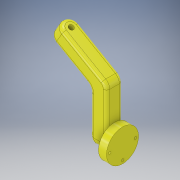
# Autodesk Inventor part: Link1
Saved by Autodesk Inventor 2019 (Build 230136000, 136)
## iProperties
Created: 2022-07-14
Part Number: Link1
Material: Generic
Document SubType Name: Modeling
Designer: zreik
Density: 1 g/cm^3
Appearance: Yellow
thickness: 10.000 mm
width: 10.000 mm
radius: 60.000 mm
Author: zreik
Autodesk Inventor part; units mm, degrees
sketch "Sketch1" plane through (0, 0, 0) normal (0, 0, 1) x (1, 0, 0)
  line L0 (54.744646, 0) -> (0, 0)
  line L1 (0, 0) -> (30, 51.961524)
  line L2 (44.744646, 0) -> (44.744646, 23.613249)
  line L3 (42.244646, 27.943376) -> (22.660998, 39.25)
  line L4 (54.744646, 0) -> (54.744646, 29.386751)
  line L5 (52.244646, 33.716878) -> (27.660998, 47.910254)
  arc A0 (44.744646, 23.613249) -> (42.244646, 27.943376) centre (39.744646, 23.613249) ccw
  arc A1 (54.744646, 29.386751) -> (52.244646, 33.716878) centre (49.744646, 29.386751) ccw
  line L6 (27.660998, 47.910254) -> (22.660998, 39.25)
  line L7 (27.660998, 47.910254) -> (52.244646, 33.716878)
  line L8 (22.660998, 39.25) -> (42.244646, 27.943376)
  line L9 (44.744646, 0) -> (54.744646, 0)
  line L10 (54.744646, 0) -> (54.744646, 29.386751)
  line L11 (44.744646, 0) -> (54.744646, 0)
  line L12 (54.744646, 0) -> (54.744646, 29.386751)
  line L13 (52.244646, 33.716878) -> (27.660998, 47.910254)
  line L14 (27.660998, 47.910254) -> (22.660998, 39.25)
  line L15 (22.660998, 39.25) -> (42.244646, 27.943376)
  line L16 (44.744646, 23.613249) -> (44.744646, 0)
  point P0 (25, 43.30127)
  point P1 (44.744646, 26.5)
  dimension "d0" = 60
  dimension "d35" = 10
  dimension "d37" = 10
  dimension "d38" = 0
  dimension "d39" = 0
  dimension "d41" = 26.5
  dimension "d42" = 25.5
  dimension "d43" = 120
  dimension "d44" = 5
  constraints: 34 end point, 9 collinear, 6 point on line, 4 point on circle, 4 tangent, 2 centre point, 2 parallel, 1 equal radius, 1 horizontal, 1 vertical
  measures "d0" angle of L1 L0
  measures "d35" distance between parallel lines of L3 L5
  measures "d37" distance between parallel lines of L4 L2
  measures "d38" distance from line of L1 L3.end
  measures "d39" distance from line of L1 L5.end
  measures "d41" distance of L2.start point (44.745, 26.5)
  measures "d42" distance of point (44.745, 26.5) L3.end
  measures "d43" angle of L2 L3
  measures "d44" radius of A0
extrude "Extrusion1" add sketch "Sketch1" along normal blind 10 contours L0 L2 A0 L3 L1 L5 A1 L4
ref_plane "Work Plane1" through (39.952822, 40.813566, 0) normal (0.5, 0.8660254, 0) x (0.8660254, -0.5, 0)
sketch "Sketch2" plane through (39.952822, 40.813566, 0) normal (0.5, 0.8660254, 0) x (0.8660254, -0.5, 0)
  circle A0 centre (-14.193376, -5) radius 5
  line L0 (-14.193376, 0) -> (-14.193376, -10)
  line L1 (14.193376, 0) -> (-14.193376, 0)
  dimension "d5" = 10
  dimension "d45" = 0
  dimension "d46" = 5
  constraints: 1 centre point
  measures "d5" diameter of A0
  measures "d45" distance from line of L0 A0.centre
  measures "d46" distance from line of L1 A0.centre
extrude "Extrusion2" add sketch "Sketch2" against normal blind 10
ref_plane "Work Plane2" through (54.744646, 0, 5) normal (1, 0, 0) x (0, 0, -1)
sketch "Sketch3" plane through (54.744646, 0, 5) normal (1, 0, 0) x (0, 0, -1)
  circle A0 centre (0, 0) radius 5
  line L0 (5, 0) -> (-5, 0)
  line L1 (-5, 0) -> (-5, 29.386751)
  point P0 (-5, 39.25)
  dimension "d10" = 10
  dimension "d47" = 0
  dimension "d48" = 5
  constraints: 1 centre point, 1 vertical alignment
  measures "d10" diameter of A0
  measures "d47" distance from line of L0 A0.centre
  measures "d48" distance from line of L1 A0.centre
extrude "Extrusion3" add sketch "Sketch3" against normal blind 10
sketch "Sketch4" plane through (34.952822, 32.153312, 0) normal (-0.5, -0.8660254, 0) x (-0.8660254, 0.5, 0)
  circle A0 centre (14.193376, -5) radius 1.5
  circle A1 centre (14.193376, -5) radius 5
  point P0 (14.193376, 0)
  point P1 (14.193376, -10)
  dimension "d15" = 3
  constraints: 1 centre point, 1 concentric
  measures "d15" diameter of A0
extrude "Extrusion4" cut sketch "Sketch4" against normal blind 50 contours A0
sketch "Sketch5" plane through (44.744646, 0, 5) normal (-1, 0, 0) x (0, 1, 0)
  circle A0 centre (0, 0) radius 1.5
  arc A1 (0, 5) -> (0, -5) centre (0, 0) ccw projected
  dimension "d18" = 3
  constraints: 1 centre point, 1 concentric
  measures "d18" diameter of A0
extrude "Extrusion5" cut sketch "Sketch5" against normal blind 50
sketch "Sketch6" plane through (34.952822, 32.153312, 0) normal (-0.5, -0.8660254, 0) x (-0.8660254, 0.5, 0)
  circle A0 centre (14.193376, -5) radius 3.5
  circle A1 centre (14.193376, -5) radius 5
  circle A2 centre (14.193376, -5) radius 1.5
  arc A3 (15.693376, -5) -> (15.693376, -5) centre (14.193376, -5) ccw
  point P0 (14.193376, 0)
  point P1 (14.193376, -10)
  dimension "d21" = 7
  dimension "d24" = 3
  constraints: 2 centre point, 1 coincident, 1 concentric
  measures "d21" diameter of A0
extrude "Extrusion6" add sketch "Sketch6" along normal blind 1.258 contours A0
chamfer "Chamfer1" distance 1 angle 45 1 edges at (25.0631, 36.4105, 5)
sketch "Sketch7" plane through (44.744646, 0, 5) normal (-1, 0, 0) x (0, 1, 0)
  circle A0 centre (0, 0) radius 1.5
  circle A1 centre (0, 0) radius 3.5
  arc A2 (1.5, 0) -> (1.5, 0) centre (0, 0) ccw projected
  point P0 (0, 5)
  dimension "d28" = 3
  dimension "d29" = 7
  constraints: 2 centre point, 1 coincident, 1 concentric
  measures "d28" diameter of A0
  measures "d29" diameter of A1
extrude "Extrusion7" add sketch "Sketch7" along normal blind 1.443
chamfer "Chamfer2" distance 1 angle 45 1 edges at (43.3016, -3.5, 5)
fillet "Fillet1" radius 2 16 edges at (23.3309, 50.4103, 5) (39.9528, 40.8136, 0) (54.0748, 31.8868, 0) (54.7446, 14.6934, 0) (54.7446, -5, 5) (54.7446, 14.6934, 10) (54.0748, 31.8868, 10) (39.9528, 40.8136, 10) (44.0748, 26.1132, 10) (44.7446, 11.8066, 10) (44.7446, -5, 5) (44.7446, 11.8066, 0) (44.0748, 26.1132, 0) (32.4528, 33.5967, 0) (18.3309, 41.75, 5) (32.4528, 33.5967, 10)
ref_plane "Work Plane3" through (0, 0, 5) normal (0, 0, 1) x (1, 0, 0)
sketch "Sketch10" plane through (0, 0, 5) normal (0, 0, 1) x (1, 0, 0)
  line L0 (54.744646, 1.5) -> (54.744646, -1.5)
  line L1 (54.744646, 0) -> (59.744646, 0)
  line L2 (59.744646, 0) -> (59.744646, 10)
  line L3 (59.744646, 10) -> (54.744646, 10)
  line L4 (54.744646, 10) -> (54.744646, 0)
  point P0 (0, 0)
  dimension "d75" = 5
  dimension "d76" = 10
  constraints: 8 end point, 2 parallel, 1 horizontal, 1 midpoint, 1 perpendicular
  measures "d75" distance of L1.start L1.end
  measures "d76" distance of L1.end L2.end
revolve "Revolution2" add sketch "Sketch10" angle 360 about axis through (54.744646, 0, 5) along (1, 0, 0)
sketch "Sketch11" plane through (59.744646, 0, 5) normal (1, 0, 0) x (0, 0, -1)
  circle A0 centre (8, 0) radius 0.8
  line L0 (5, 0) -> (3, 0) projected
  circle A1 centre (0, 0) radius 1.5 projected
  circle A2 centre (0, -8) radius 0.8
  circle A3 centre (-8, 0) radius 0.8
  dimension "d78" = 1.6
  dimension "d79" = 0
  dimension "d80" = 8
  dimension "d83" = 180
  constraints: 3 centre point, 5 other
  measures "d78" diameter of A0
  measures "d79" distance from line of L0 A0.centre
  measures "d80" distance of A1.centre A0.centre
extrude "Extrusion9" cut sketch "Sketch11" against normal up to next contours A0 | A2 | A3
equation "\"d35\" = thickness"
equation "\"d37\" = thickness"
equation "\"d3\" = width"
equation "\"d5\" = width"
equation "\"d46\" = 0.5 * width"
equation "\"d8\" = thickness"
equation "\"d10\" = width"
equation "\"d48\" = 0.5 * width"
equation "\"d13\" = thickness"
equation "\"thickness\" = 10"
equation "\"width\" = 10"
equation "\"radius\" = 60"
body "Solid1"
